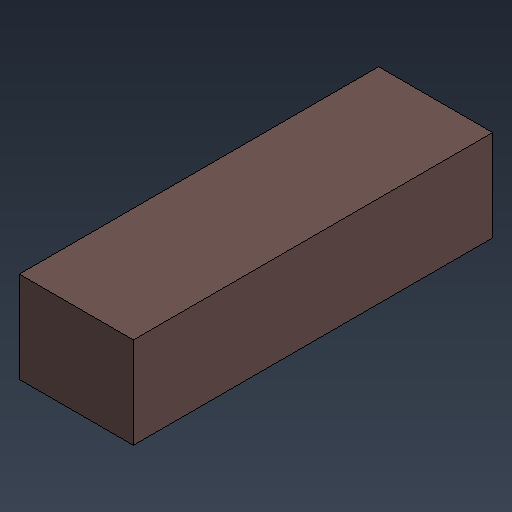
# Autodesk Inventor part: 2s450mah
Saved by Autodesk Inventor 2026.2 (Build 302298010, 298A)
## iProperties
Created: 2026-03-09
Part Number: 2s450mah
Material: Generic
Document SubType Name: Modeling
Designer: szymo
Density: 2.3523 g/cm^3
Appearance: Default(3)
Mass: 50 g
Surface Area: 54.1881 cm^2
Volume: 21.2558 cm^3
Author: szymo
Autodesk Inventor part; units mm, degrees
ref_plane "YZ Plane" through (0, 0, 0) normal (1, 0, 0) x (0, 1, 0)
ref_plane "XZ Plane" through (0, 0, 0) normal (0, 1, 0) x (-1, 0, 0)
ref_plane "XY Plane" through (0, 0, 0) normal (0, 0, 1) x (1, 0, 0)
sketch "Sketch1" plane through (0, 0, 0) normal (0, 1, 0) x (-1, 0, 0)
  line L0 (0, 0) -> (-20, 0)
  line L1 (-20, 0) -> (-20, -63)
  line L2 (-20, -63) -> (0, -63)
  line L3 (0, -63) -> (0, 0)
  dimension "d0" = 20
  dimension "d1" = 63
  constraints: 8 end point, 2 parallel, 1 horizontal, 1 perpendicular
  measures "d0" distance of L2.end L1.end
  measures "d1" distance of L0.end L1.end
extrude "Extrusion1" add sketch "Sketch1" along normal blind 16
body "Solid1"
